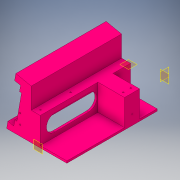
# Autodesk Inventor part: CPURightTwo
Saved by Autodesk Inventor 2019 (Build 230136000, 136)
## iProperties
Created: 2019-01-04
Part Number: CPURightTwo
Material: Generic
Document SubType Name: Modeling
Designer: james
Density: 1 g/cm^3
Appearance: Default(1)
Author: james
Autodesk Inventor part; units mm, degrees
ref_plane "YZ Plane" through (0, 0, 0) normal (1, 0, 0) x (0, 1, 0)
ref_plane "XZ Plane" through (0, 0, 0) normal (0, 1, 0) x (-1, 0, 0)
ref_plane "XY Plane" through (0, 0, 0) normal (0, 0, 1) x (1, 0, 0)
sketch "Sketch1" plane through (0, 0, 0) normal (0, 1, 0) x (-1, 0, 0)
  line L0 (45.7123, 188.7629) -> (-21.5977, 188.7629)
  line L1 (-21.5977, 188.7629) -> (-21.5977, -39.8371)
  line L2 (-21.5977, -39.8371) -> (45.7123, -39.8371)
  line L3 (45.7123, -39.8371) -> (45.7123, 188.7629)
  point P0 (0, 0)
  dimension "d0" = 228.6
  dimension "d1" = 67.31
  constraints: 8 end point, 2 parallel, 1 horizontal, 1 perpendicular
  measures "d0" distance of L0.end L1.end
  measures "d1" distance of L1.end L2.end
extrude "Extrusion1" add sketch "Sketch1" along normal blind 5.08
sketch "Sketch53" plane through (21.5977, 0, 188.7629) normal (0, 0, 1) x (1, 0, 0)
  line L0 (-67.31, 71.12) -> (-67.31, 5.08) projected
  line L1 (-72.39, 71.12) -> (-67.31, 71.12) projected
  line L2 (-67.31, 71.12) -> (-95.25, 71.12)
  line L3 (-95.25, 71.12) -> (-95.25, 66.04)
  line L4 (-95.25, 66.04) -> (-67.31, 66.04)
  line L5 (-67.31, 66.04) -> (-67.31, 71.12)
  line L6 (-98.425, 66.04) -> (-111.125, 66.04) projected
  line L7 (-111.125, 66.04) -> (-111.125, 71.12) projected
  point P0 (-21.5977, 0)
  point P1 (-125.73, 66.04)
  dimension "d180" = 0
  dimension "d255" = 27.94
  constraints: 8 end point, 2 parallel, 1 horizontal, 1 perpendicular
  measures "d180" distance between parallel lines of L4 L6
  measures "d255" distance of L0.start L2.end
extrude "Extrusion39" add sketch "Sketch53" against normal blind 228.6
ref_plane "Work Plane6" through (-45.7123, 71.12, -34.7571) normal (0, 1, 0) x (1, 0, 0)
sketch "Sketch60" plane through (21.5977, 0, 188.7629) normal (0, 0, 1) x (1, 0, 0)
  line L0 (-67.31, 0) -> (0, 0) projected
  line L1 (-147.32, 0) -> (-152.4, 0)
  line L2 (-147.32, 0) -> (-117.3637, 169.8909)
  line L3 (-98.425, 5.08) -> (-98.425, 71.12) projected
  line L4 (-152.4, 0) -> (-122.4437, 169.8909)
  line L5 (-117.3637, 169.8909) -> (-122.4437, 169.8909)
  point P0 (-21.5977, 0)
  point P1 (-72.39, 0)
  point P2 (-98.425, 66.04)
  dimension "d223" = 5.08
  dimension "d224" = 0
  dimension "d225" = 152.4
  dimension "d226" = 10
  dimension "d227" = 10
  constraints: 8 end point, 2 horizontal
  measures "d223" distance of L1.start L1.end
  measures "d224" distance between parallel lines of L0 L1
  measures "d225" distance of L0.end L1.end
  measures "d226" angle of L2 L3
  measures "d227" angle of L3 L4
extrude "Extrusion42" add sketch "Sketch60" against normal blind 228.6
ref_plane "Work Plane8" through (-50.7923, 0, 188.7629) normal (0, 0, 1) x (1, 0, 0)
sketch "Sketch66" plane through (-50.7923, 0, 188.7629) normal (0, 0, 1) x (1, 0, 0)
  line L0 (5.08, 71.12) -> (-22.86, 71.12) projected
  line L1 (-22.86, 66.04) -> (0, 66.04) projected
  line L2 (-17.78, 66.04) -> (-22.86, 66.04)
  line L3 (-22.86, 66.04) -> (-22.86, 162.1783)
  line L4 (-22.86, 162.1783) -> (-17.78, 162.1783)
  line L5 (-17.78, 162.1783) -> (-17.78, 66.04)
  line L6 (5.08, 71.12) -> (5.08, 5.08) projected
  point P0 (50.7923, 0)
  point P1 (-62.3896, 71.12)
  point P2 (-63.2854, 66.04)
  dimension "d245" = 5.08
  dimension "d252" = 22.86
  constraints: 8 end point, 2 parallel, 1 horizontal, 1 perpendicular, 1 point on line
  measures "d245" distance between parallel lines of L3 L5
  measures "d252" distance between parallel lines of L5 L6
extrude "Extrusion48" add sketch "Sketch66" against normal blind 228.6
ref_plane "Work Plane4" through (21.5977, 71.12, -58.8871) normal (1, 0, 0) x (0, 0, -1)
ref_plane "Work Plane5" through (21.5977, 66.04, -58.8871) normal (0, 0, 1) x (1, 0, 0)
ref_plane "Work Plane9" through (-50.7923, 0, 188.7629) normal (0, 0, 1) x (1, 0, 0)
sketch "Sketch76" plane through (-50.7923, 0, 188.7629) normal (0, 0, 1) x (1, 0, 0)
  line L0 (72.39, 105.3084) -> (-17.78, 124.113) projected
  line L1 (-22.86, 125.1725) -> (-51.7947, 131.2067) projected
  line L2 (-56.6945, 132.2285) -> (-81.3081, 137.3616) projected
  line L3 (-81.3081, 137.3616) -> (72.39, 105.3084)
  line L4 (72.39, 105.3084) -> (72.39, 181.982)
  line L5 (72.39, 181.982) -> (-81.3081, 181.982)
  line L6 (-81.3081, 137.3616) -> (-81.3081, 181.982)
  point P0 (50.7923, 0)
  constraints: 8 end point, 2 vertical, 1 perpendicular
extrude "Extrusion56" cut sketch "Sketch76" against normal blind 312.7375
sketch "Sketch89" plane through (21.5977, 0, 188.7629) normal (0, 0, 1) x (1, 0, 0)
  line L0 (-67.31, 71.12) -> (-90.17, 71.12) projected
  line L1 (-67.31, 66.04) -> (-67.31, 71.12) projected
  line L2 (-67.31, 71.12) -> (-72.39, 71.12)
  line L3 (-72.39, 71.12) -> (-72.39, 0)
  line L4 (-72.39, 0) -> (-67.31, 0)
  line L5 (-67.31, 0) -> (-67.31, 71.12)
  point P0 (-21.5977, 0)
  dimension "d326" = 5.08
  constraints: 8 end point, 2 parallel, 1 horizontal, 1 perpendicular
  measures "d326" distance between parallel lines of L5 L3
extrude "Extrusion65" add sketch "Sketch89" against normal blind 228.6
sketch "Sketch90" plane through (21.5977, 0, 188.7629) normal (0, 0, 1) x (1, 0, 0)
  line L0 (-152.4, 0) -> (-129.0845, 132.2285) projected
  line L1 (-124.1847, 131.2067) -> (-129.0845, 132.2285) projected
  line L2 (-124.1847, 131.2067) -> (-147.32, 0) projected
  line L3 (-90.17, 124.113) -> (-95.25, 125.1725) projected
  line L4 (-90.17, 124.113) -> (-90.17, 71.12) projected
  line L5 (-129.0845, 132.2285) -> (-90.17, 124.113)
  line L6 (-90.17, 124.113) -> (-90.17, 118.9238)
  line L7 (-90.17, 118.9238) -> (-129.9671, 127.2233)
  line L8 (-129.0845, 132.2285) -> (-129.9671, 127.2233)
  point P0 (-21.5977, 0)
  dimension "d329" = 5.08
  constraints: 8 end point, 2 point on line, 1 parallel
  measures "d329" distance between parallel lines of L5 L7
extrude "Extrusion66" add sketch "Sketch90" against normal blind 228.6
sketch "Sketch91" plane through (-45.7123, 5.08, 188.7629) normal (0, 0, 1) x (1, 0, 0)
  line L0 (0, 0) -> (0, 66.04) projected
  line L1 (-5.08, -5.08) -> (67.31, -5.08) projected
  line L2 (-85.09, -5.08) -> (-61.7745, 127.1485) projected
  line L3 (-80.01, -5.08) -> (-85.09, -5.08) projected
  line L4 (0, 66.04) -> (-22.86, 66.04) projected
  line L5 (-22.86, 119.033) -> (-22.86, 66.04) projected
  line L6 (-22.86, 119.033) -> (-61.7745, 127.1485) projected
  line L7 (0, 66.04) -> (0, 0) projected
  line L8 (0, 66.04) -> (0, -5.08)
  line L9 (67.31, -5.08) -> (-5.08, -5.08) projected
  line L10 (-85.09, -5.08) -> (0, -5.08)
  line L11 (-80.01, -5.08) -> (-85.09, -5.08) projected
  line L12 (-61.7745, 127.1485) -> (-22.86, 119.033) projected
  line L13 (-85.09, -5.08) -> (-61.7745, 127.1485)
  line L14 (-61.7745, 127.1485) -> (-22.86, 119.033)
  line L15 (-22.86, 119.033) -> (-22.86, 66.04) projected
  line L16 (-22.86, 119.033) -> (-22.86, 66.04)
  line L17 (-22.86, 66.04) -> (0, 66.04) projected
  line L18 (-22.86, 66.04) -> (0, 66.04)
  point P0 (45.7123, -5.08)
  constraints: 12 end point, 2 collinear, 2 perpendicular
extrude "Extrusion67" add sketch "Sketch91" against normal blind 5.08
sketch "Sketch92" plane through (21.5977, 5.08, -39.8371) normal (0, 0, -1) x (-1, 0, 0)
  line L0 (67.31, 66.04) -> (67.31, 0) projected
  line L1 (0, -5.08) -> (72.39, -5.08) projected
  line L2 (152.4, -5.08) -> (129.0845, 127.1485) projected
  line L3 (129.0845, 127.1485) -> (90.17, 119.033) projected
  line L4 (90.17, 119.033) -> (90.17, 66.04) projected
  line L5 (90.17, 66.04) -> (67.31, 66.04) projected
  line L6 (152.4, -5.08) -> (129.0845, 127.1485) projected
  line L7 (129.0845, 127.1485) -> (90.17, 119.033)
  line L8 (90.17, 119.033) -> (90.17, 66.04)
  line L9 (90.17, 66.04) -> (67.31, 66.04)
  line L10 (67.31, 66.04) -> (67.31, -5.08)
  line L11 (129.0845, 127.1485) -> (152.4, -5.08)
  line L12 (152.4, -5.08) -> (67.31, -5.08)
  line L13 (152.4, -5.08) -> (0, -5.08) projected
  point P0 (21.5977, -5.08)
  constraints: 12 end point, 3 collinear, 1 perpendicular
extrude "Extrusion68" add sketch "Sketch92" against normal blind 5.08
sketch "Sketch93" plane through (21.5977, 5.08, -39.8371) normal (0, 0, -1) x (-1, 0, 0)
  line L0 (67.31, 66.04) -> (67.31, 0) projected
  line L1 (0, -5.08) -> (152.4, -5.08) projected
  point P0 (21.5977, -5.08)
  point P1 (118.11, 20.32)
  point P2 (118.11, 45.72)
  dimension "d336" = 50.8
  dimension "d337" = 50.8
  dimension "d338" = 25.4
  dimension "d339" = 25.4
  measures "d336" distance from line of L0 point (118.11, 20.32)
  measures "d337" distance from line of L0 point (118.11, 45.72)
  measures "d338" distance from line of L1 point (118.11, 20.32)
  measures "d339" distance of point (118.11, 45.72) point (118.11, 20.32)
hole "Hole14" at (-96.5123, 25.4, -39.8371) at (-96.5123, 50.8, -39.8371) direction (0, 0, 1) diameter 3.302 end through all
sketch "Sketch94" plane through (-45.7123, 71.12, 188.7629) normal (0, 1, 0) x (1, 0, 0)
  line L0 (0, 0) -> (0, 228.6) projected
  line L1 (-22.86, 228.6) -> (-22.86, 0) projected
  line L2 (-22.86, 228.6) -> (0, 228.6) projected
  line L3 (67.31, 0) -> (67.31, 228.6) projected
  line L4 (-22.86, 228.6) -> (-22.86, 0) projected
  line L5 (-22.86, 146.05) -> (67.31, 146.05)
  line L6 (67.31, 146.05) -> (67.31, 184.15)
  line L7 (67.31, 184.15) -> (-22.86, 184.15)
  line L8 (-22.86, 184.15) -> (-22.86, 146.05)
  point P0 (45.7123, 188.7629)
  dimension "d347" = 44.45
  dimension "d348" = 38.1
  constraints: 8 end point, 2 parallel, 2 point on line, 1 horizontal, 1 perpendicular
  measures "d347" distance between parallel lines of L7 L2
  measures "d348" distance between parallel lines of L5 L7
extrude "Extrusion69" add sketch "Sketch94" against normal blind 5.08 contours L5 L1 L7 L0 | L0 L7 L3 L5
sketch "Sketch95" plane through (21.5977, 71.12, 42.7129) normal (1, 0, 0) x (0, 0, -1)
  line L0 (0, 0) -> (38.1, 0) projected
  line L1 (38.1, 0) -> (38.1, -5.08) projected
  line L2 (0, 0) -> (0, -5.08) projected
  line L3 (-146.05, -71.12) -> (82.55, -71.12) projected
  line L4 (-140.97, -71.12) -> (77.47, -71.12) projected
  line L5 (0, 0) -> (5.08, 0)
  line L6 (5.08, 0) -> (5.08, -71.12)
  line L7 (5.08, -71.12) -> (0, -71.12)
  line L8 (0, -71.12) -> (0, 0)
  line L9 (38.1, 0) -> (33.02, 0)
  line L10 (33.02, 0) -> (33.02, -71.12)
  line L11 (33.02, -71.12) -> (38.1, -71.12)
  line L12 (38.1, -71.12) -> (38.1, 0)
  point P0 (42.7129, -71.12)
  dimension "d351" = 5.08
  dimension "d352" = 5.08
  constraints: 16 end point, 4 parallel, 2 horizontal, 2 perpendicular, 2 point on line
  measures "d351" distance between parallel lines of L10 L12
  measures "d352" distance between parallel lines of L8 L6
extrude "Extrusion70" add sketch "Sketch95" against normal blind 69.5325 contours L0 L6 L3 L8 L2 | L0 L1 L12 L3 L10
sketch "Sketch96" plane through (21.5977, 0, 188.7629) normal (1, 0, 0) x (0, 0, -1)
  line L0 (179.07, 66.04) -> (179.07, 5.08) projected
  line L1 (151.13, 5.08) -> (151.13, 66.04) projected
  line L2 (0, 0) -> (228.6, 0) projected
  line L3 (5.08, 0) -> (223.52, 0) projected
  line L4 (151.13, 5.08) -> (179.07, 5.08)
  line L5 (179.07, 5.08) -> (179.07, 0)
  line L6 (179.07, 0) -> (151.13, 0)
  line L7 (151.13, 0) -> (151.13, 5.08)
  point P0 (188.7629, 0)
  constraints: 8 end point, 2 parallel, 1 horizontal, 1 perpendicular, 1 point on line
extrude "Extrusion71" cut sketch "Sketch96" against normal blind 66.3575
sketch "Sketch97" plane through (21.5977, 5.08, 4.6129) normal (1, 0, 0) x (0, 0, -1)
  line L0 (-38.1, 66.04) -> (0, 66.04) projected
  line L1 (0, 66.04) -> (0, 0) projected
  line L2 (-38.1, 66.04) -> (-38.1, 0) projected
  line L3 (-5.08, -5.08) -> (-33.02, -5.08) projected
  line L4 (-179.07, -5.08) -> (39.37, -5.08) projected
  line L5 (-38.1, 66.04) -> (0, 66.04)
  line L6 (0, 66.04) -> (0, -5.08)
  line L7 (0, -5.08) -> (-38.1, -5.08)
  line L8 (-38.1, -5.08) -> (-38.1, 66.04)
  point P0 (4.6129, -5.08)
  constraints: 8 end point, 2 parallel, 1 horizontal, 1 perpendicular, 1 point on line
extrude "Extrusion72" add sketch "Sketch97" against normal blind 5.08
sketch "Sketch101" plane through (-45.7123, 5.08, 183.6829) normal (0, 0, -1) x (-1, 0, 0)
  line L0 (5.08, 60.96) -> (27.94, 60.96) projected
  line L1 (5.08, 60.96) -> (5.08, -5.08) projected
  line L2 (5.08, -5.08) -> (5.08, 60.96) projected
  line L3 (5.08, -5.08) -> (5.08, 60.96) projected
  line L4 (5.08, 60.96) -> (5.08, 46.5843)
  line L5 (5.08, 46.5843) -> (27.94, 60.96)
  line L6 (27.8708, 61.07) -> (5.08, 60.96)
  point P0 (-45.7123, -5.08)
  constraints: 6 end point, 1 point on line
extrude "Extrusion73" add sketch "Sketch101" along normal blind 219.3925
sketch "Sketch98" plane through (21.5977, 0, 188.7629) normal (1, 0, 0) x (0, 0, -1)
  line L0 (184.15, 71.12) -> (184.15, 5.08) projected
  line L1 (0, 0) -> (228.6, 0) projected
  point P0 (188.7629, 0)
  point P1 (165.1, 25.4)
  dimension "d359" = 19.05
  dimension "d360" = 25.4
  measures "d359" distance from line of point (165.1, 25.4) L0
  measures "d360" distance from line of L1 point (165.1, 25.4)
hole "Hole15" at (21.5977, 25.4, 23.6629) direction (-1, 0, 0) diameter 3.302 depth 25.4 tip angle 118.188
sketch "Sketch99" plane through (-68.5723, 71.12, 188.7629) normal (0, 1, 0) x (1, 0, 0)
  line L0 (22.86, 0) -> (22.86, 146.05) projected
  line L1 (22.86, 0) -> (0, 0) projected
  point P0 (68.5723, 188.7629)
  point P1 (10.7696, 12.7)
  point P2 (10.7696, 88.9)
  dimension "d368" = 12.0904
  dimension "d369" = 12.0904
  dimension "d370" = 12.7
  dimension "d371" = 76.2
  measures "d368" distance from line of L0 point (10.77, 88.9)
  measures "d369" distance from line of L0 point (10.77, 12.7)
  measures "d370" distance from line of L1 point (10.77, 12.7)
  measures "d371" distance of point (10.77, 88.9) point (10.77, 12.7)
hole "Hole16" at (-57.8027, 71.12, 176.0629) at (-57.8027, 71.12, 99.8629) direction (0, -1, 0) diameter 3.302 depth 25.4 tip angle 118.188
sketch "Sketch100" plane through (-68.5723, 71.12, 188.7629) normal (0, 1, 0) x (1, 0, 0)
  line L0 (22.86, 146.05) -> (90.17, 146.05) projected
  line L1 (90.17, 184.15) -> (22.86, 184.15) projected
  line L2 (90.17, 146.05) -> (90.17, 184.15) projected
  point P0 (68.5723, 188.7629)
  point P1 (77.47, 155.575)
  point P2 (77.47, 174.625)
  dimension "d379" = 9.525
  dimension "d380" = 9.525
  dimension "d381" = 12.7
  dimension "d382" = 12.7
  measures "d379" distance from line of L0 point (77.47, 155.575)
  measures "d380" distance from line of L1 point (77.47, 174.625)
  measures "d381" distance from line of L2 point (77.47, 174.625)
  measures "d382" distance from line of L2 point (77.47, 155.575)
hole "Hole17" at (8.8977, 71.12, 33.1879) at (8.8977, 71.12, 14.1379) direction (0, -1, 0) diameter 3.302 depth 25.4 tip angle 118.188
sketch "Sketch102" plane through (-130.8023, 0, -39.8371) normal (-0.9848078, 0.1736482, 0) x (0, 0, 1)
  line L0 (68.58, 116.84) -> (228.6, 116.84)
  line L1 (228.6, 116.84) -> (228.6, 17.78)
  line L2 (228.6, 17.78) -> (68.58, 17.78)
  line L3 (68.58, 17.78) -> (68.58, 116.84)
  line L4 (228.6, 0) -> (228.6, 134.2684) projected
  line L5 (228.6, 0) -> (0, 0) projected
  point P0 (39.8371, 22.7136)
  dimension "d392" = 0
  dimension "d393" = 160.02
  dimension "d394" = 17.78
  dimension "d395" = 99.06
  constraints: 8 end point, 2 parallel, 1 horizontal, 1 perpendicular
  measures "d392" distance between parallel lines of L4 L1
  measures "d393" distance between parallel lines of L1 L3
  measures "d394" distance between parallel lines of L5 L2
  measures "d395" distance between parallel lines of L0 L2
extrude "Extrusion74" cut sketch "Sketch102" against normal blind 15.24
sketch "Sketch103" plane through (-45.7123, 5.08, 183.6829) normal (0, 0, -1) x (-1, 0, 0)
  line L0 (77.0757, 11.5612) -> (66.9941, 9.7835) projected
  line L1 (66.9941, 9.7835) -> (49.7925, 107.3385) projected
  line L2 (49.7925, 107.3385) -> (59.8741, 109.1162) projected
  arc A0 (77.0757, 11.5612) -> (77.0757, 11.5612) centre (74.5553, 11.1167) ccw
  line L3 (77.0757, 11.5612) -> (77.7373, 7.809)
  line L4 (66.9941, 9.7835) -> (82.0025, 12.4299) projected
  line L5 (77.7373, 7.809) -> (63.9035, 5.3698)
  line L6 (63.9035, 5.3698) -> (45.3788, 110.4291)
  line L7 (45.3788, 110.4291) -> (59.2125, 112.8683)
  line L8 (57.7573, 121.1215) -> (59.8741, 109.1162) projected
  line L9 (59.8741, 109.1162) -> (59.2125, 112.8683)
  line L10 (59.8741, 109.1162) -> (49.7925, 107.3385)
  line L11 (49.7925, 107.3385) -> (66.9941, 9.7835)
  line L12 (49.7925, 107.3385) -> (66.9941, 9.7835) projected
  line L13 (66.9941, 9.7835) -> (77.0757, 11.5612)
  point P0 (-45.7123, -5.08)
  dimension "d398" = 3.81
  dimension "d399" = 3.81
  dimension "d400" = 3.81
  constraints: 16 end point, 4 perpendicular, 4 point on line, 3 collinear, 2 point on circle, 1 centre point
  measures "d398" distance between parallel lines of L5 L0
  measures "d399" distance between parallel lines of L6 L1
  measures "d400" distance between parallel lines of L2 L7
extrude "Extrusion75" add sketch "Sketch103" along normal blind 164.465 contours A0 L0 | L3 L5 L6 L7 L8 L2 L1 L0 A0 picked at (75.381, 10.3626)
sketch "Sketch104" plane through (-127.7148, 17.5099, 28.7429) normal (0, 0, 1) x (0.9848078, -0.1736482, 0)
  line L0 (15.24, 99.06) -> (15.24, 0) projected
  line L1 (15.24, 0) -> (15.24, 99.06) projected
  line L2 (0, 0) -> (0, 99.06) projected
  line L3 (0, 99.06) -> (15.24, 99.06)
  line L4 (15.24, 99.06) -> (15.24, 0)
  line L5 (15.24, 0) -> (0, 0)
  line L6 (0, 0) -> (0, 99.06)
  point P0 (128.8151, 4.9336)
  constraints: 8 end point, 2 parallel, 1 horizontal, 1 perpendicular
extrude "Extrusion76" add sketch "Sketch104" against normal blind 5.08
sketch "Sketch105" plane through (-45.7123, 5.08, 188.7629) normal (1, 0, 0) x (0, 0, -1)
  line L0 (36.4741, 32.3893) -> (122.561, 33.5073) construction
  line L1 (36.7461, 11.4511) -> (122.8329, 12.5691)
  line L2 (122.2891, 54.4455) -> (36.2022, 53.3275)
  arc A0 (36.2022, 53.3275) -> (36.7461, 11.4511) centre (36.4741, 32.3893) ccw
  arc A1 (122.8329, 12.5691) -> (122.2891, 54.4455) centre (122.561, 33.5073) ccw
  point P0 (188.7629, -5.08)
  point P1 (79.5176, 32.9483)
  constraints: 8 end point, 4 point on circle, 4 tangent, 2 centre point, 1 midpoint, 1 parallel
extrude "Extrusion77" cut sketch "Sketch105" against normal blind 5.08
sketch "Sketch106" plane through (-115.7938, -2.6464, -39.8371) normal (-0.9848078, 0.1736482, 0) x (0, 0, 1)
  line L0 (228.6, 116.84) -> (228.6, 17.78) projected
  line L1 (83.82, 33.02) -> (228.6, 33.02)
  line L2 (228.6, 33.02) -> (228.6, 101.6)
  line L3 (228.6, 101.6) -> (83.82, 101.6)
  line L4 (83.82, 101.6) -> (83.82, 33.02)
  line L5 (228.6, 17.78) -> (68.58, 17.78) projected
  line L6 (68.58, 116.84) -> (228.6, 116.84) projected
  line L7 (68.58, 17.78) -> (68.58, 116.84) projected
  point P0 (39.8371, 22.7136)
  dimension "d407" = 15.24
  dimension "d408" = 15.24
  dimension "d409" = 15.24
  constraints: 8 end point, 2 parallel, 1 horizontal, 1 perpendicular, 1 point on line
  measures "d407" distance between parallel lines of L1 L5
  measures "d408" distance between parallel lines of L6 L3
  measures "d409" distance between parallel lines of L7 L4
extrude "Extrusion78" cut sketch "Sketch106" against normal blind 5.08 contours L0 L1 L4 L3
sketch "Sketch107" plane through (21.5977, 5.08, -39.8371) normal (0, 0, -1) x (-1, 0, 0)
  circle A0 centre (113.0331, 71.9081) radius 12.7
  line L0 (152.4, -5.08) -> (129.0845, 127.1485) projected
  line L1 (129.0845, 127.1485) -> (90.17, 119.033) projected
  point P0 (21.5977, -5.08)
  dimension "d412" = 25.4
  dimension "d413" = 25.4
  dimension "d414" = 50.8
  constraints: 1 centre point
  measures "d412" diameter of A0
  measures "d413" distance from line of L0 A0.centre
  measures "d414" distance from line of L1 A0.centre
extrude "Extrusion79" cut sketch "Sketch107" against normal blind 25.4
sketch "Sketch108" plane through (-123.4496, 12.889, 19.2179) normal (-0.1736482, -0.9848078, 0) x (0.9848078, -0.1736482, 0)
  line L0 (14.0472, 164.465) -> (14.0472, 0) projected
  line L1 (0, 0) -> (10.2372, 0) projected
  line L2 (14.0472, 164.465) -> (0, 164.465)
  line L3 (0, 164.465) -> (0, 0)
  line L4 (0, 0) -> (14.0472, 0)
  line L5 (14.0472, 0) -> (14.0472, 164.465)
  point P0 (123.8123, -19.2179)
  constraints: 8 end point, 2 parallel, 1 horizontal, 1 perpendicular
extrude "Extrusion80" add sketch "Sketch108" along normal blind 25.4
sketch "Sketch109" plane through (-45.7123, 5.08, 188.7629) normal (0, 0, 1) x (1, 0, 0)
  line L0 (-85.09, -5.08) -> (67.31, -5.08) projected
  line L1 (-85.09, -5.08) -> (-56.137, -5.08)
  line L2 (-56.137, -5.08) -> (-56.137, -26.0107)
  line L3 (-56.137, -26.0107) -> (-85.09, -26.0107)
  line L4 (-85.09, -26.0107) -> (-85.09, -5.08)
  point P0 (45.7123, -5.08)
  constraints: 8 end point, 2 parallel, 1 horizontal, 1 perpendicular
extrude "Extrusion81" cut sketch "Sketch109" against normal blind 192.0875
equation "\"d2\" = WallWidth"
equation "\"d223\" = WallWidth"
equation "\"d245\" = WallWidth"
equation "\"d326\" = WallWidth"
equation "\"d329\" = WallWidth"
equation "\"d332\" = WallWidth"
equation "\"d334\" = WallWidth"
equation "\"d349\" = WallWidth"
equation "\"d351\" = WallWidth"
equation "\"d352\" = WallWidth"
equation "\"d357\" = WallWidth"
equation "\"DSLength\" = 1371.6"
equation "\"DSWidth\" = 304.8"
equation "\"DCDeckHeight\" = 76.2"
equation "\"WallWidth\" = 5.08"
equation "\"EdgeAngle\" = 10deg"
equation "\"LengthCuts\" = 152.4"
equation "\"WidthCuts\" = 50.8"
equation "\"PartLength\" = 228.6"
equation "\"PartWidth\" = 152.4"
equation "\"BoltHoldDiam\" = 6.35"
equation "\"ControlPlateLength\" = 228.6"
equation "\"ControlPlateWidth\" = 228.6"
equation "\"ControlPlateShelfLength\" = 19.05"
equation "\"ControlHoleLength\" = 190.5"
equation "\"ControlHoleWidth\" = 190.5"
equation "\"ControlHoleFromSide\" = 63.5"
equation "\"ControlHoleBoltHoleMid\" = 9.525"
equation "\"CPDeckHeight\" = 71.12"
equation "\"CPFromSide\" = 63.5"
equation "\"CPFromBack\" = 63.5"
equation "\"DU1CHWidth\" = 69.85"
equation "\"DU1CHLength\" = 146.05"
equation "\"ControlPlateScrewLength\" = 76.2"
equation "\"DSBackHeight\" = 127"
equation "\"BackShelf\" = 25.4"
equation "\"MainAngle\" = 168.22deg"
equation "\"CPDWidthHole\" = 120.65"
equation "\"CPDLengthHole\" = 146.05"
equation "\"DownBackHeight\" = 130.7084"
body "Solid1"
